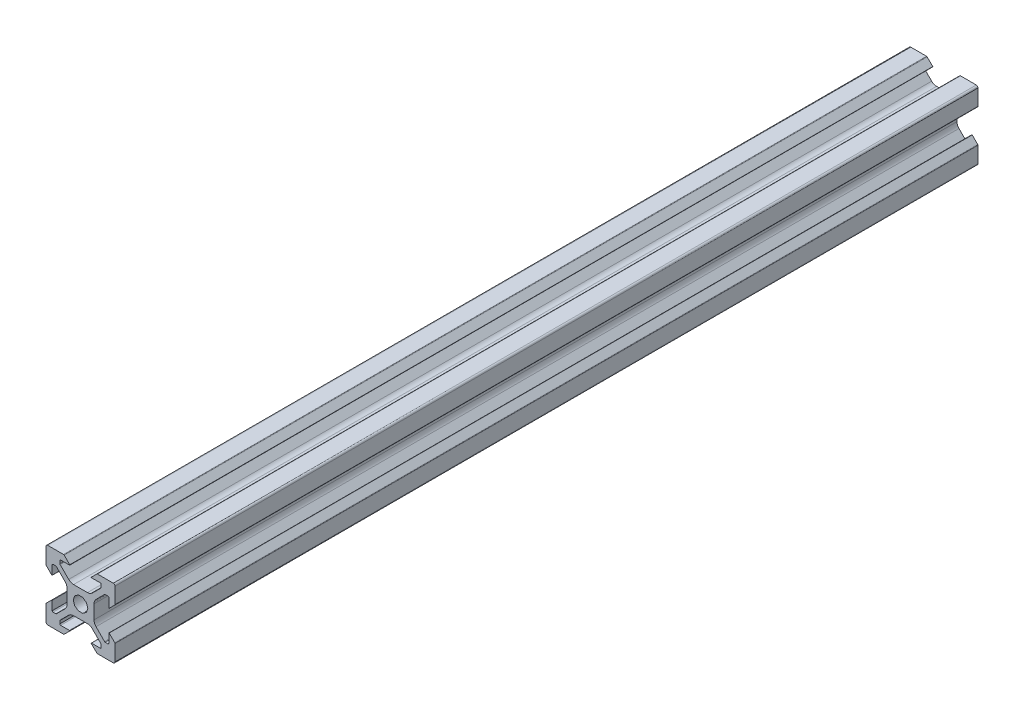
# Autodesk Inventor part: в_профиль 2020
Saved by Autodesk Inventor 2024.2 (Build 282272000, 272)
## iProperties
Created: 2026-01-28
Part Number: в_профиль 2020
Material: Типовые
Document SubType Name: Modeling
Designer: Zakhar
Density: 1 g/cm^3
Appearance: По умолчанию
Author: Zakhar
Autodesk Inventor part; units mm, degrees
ref_plane "YZ Plane" through (0, 0, 0) normal (1, 0, 0) x (0, 1, 0)
ref_plane "XZ Plane" through (0, 0, 0) normal (0, 1, 0) x (-1, 0, 0)
ref_plane "XY Plane" through (0, 0, 0) normal (0, 0, 1) x (1, 0, 0)
ref_plane "РабПлоскость1" through (93.2162, -29.7513, -35.544) normal (0, 0, 1) x (1, 0, 0)
sketch "Эскиз1" plane through (93.2162, -29.7513, -35.544) normal (0, 0, 1) x (1, 0, 0)
  line L0 (3.9, -2.0109) -> (3.9, 2.0109) projected
  arc A0 (4.4858, 3.4251) -> (3.9, 2.0109) centre (5.9, 2.0109) ccw projected
  line L1 (4.4858, 3.4251) -> (6.9874, 5.9268) projected
  arc A1 (7.1642, 6) -> (6.9874, 5.9268) centre (7.1642, 5.75) ccw projected
  line L2 (7.1642, 6) -> (7.95, 6) projected
  arc A2 (8.2, 5.75) -> (7.95, 6) centre (7.95, 5.75) ccw projected
  line L3 (8.2, 5.75) -> (8.2, 3.169) projected
  arc A3 (8.2, 3.169) -> (8.3195, 3.1195) centre (8.27, 3.169) ccw projected
  line L4 (8.3195, 3.1195) -> (9.9268, 4.7268) projected
  arc A4 (9.9268, 4.7268) -> (10, 4.9036) centre (9.75, 4.9036) ccw projected
  line L5 (10, 4.9036) -> (10, 9.5) projected
  arc A5 (10, 9.5) -> (9.5, 10) centre (9.5, 9.5) ccw projected
  line L6 (9.5, 10) -> (4.9036, 10) projected
  arc A6 (4.9036, 10) -> (4.7268, 9.9268) centre (4.9036, 9.75) ccw projected
  line L7 (4.7268, 9.9268) -> (3.1195, 8.3195) projected
  arc A7 (3.1195, 8.3195) -> (3.169, 8.2) centre (3.169, 8.27) ccw projected
  line L8 (3.169, 8.2) -> (5.75, 8.2) projected
  arc A8 (6, 7.95) -> (5.75, 8.2) centre (5.75, 7.95) ccw projected
  line L9 (6, 7.95) -> (6, 7.1642) projected
  arc A9 (5.9268, 6.9874) -> (6, 7.1642) centre (5.75, 7.1642) ccw projected
  line L10 (5.9268, 6.9874) -> (3.4251, 4.4858) projected
  arc A10 (2.0109, 3.9) -> (3.4251, 4.4858) centre (2.0109, 5.9) ccw projected
  line L11 (2.0109, 3.9) -> (-2.0109, 3.9) projected
  arc A11 (-3.4251, 4.4858) -> (-2.0109, 3.9) centre (-2.0109, 5.9) ccw projected
  line L12 (-3.4251, 4.4858) -> (-5.9268, 6.9874) projected
  arc A12 (-6, 7.1642) -> (-5.9268, 6.9874) centre (-5.75, 7.1642) ccw projected
  line L13 (-6, 7.1642) -> (-6, 7.95) projected
  arc A13 (-5.75, 8.2) -> (-6, 7.95) centre (-5.75, 7.95) ccw projected
  line L14 (-5.75, 8.2) -> (-3.169, 8.2) projected
  arc A14 (-3.169, 8.2) -> (-3.1195, 8.3195) centre (-3.169, 8.27) ccw projected
  line L15 (-3.1195, 8.3195) -> (-4.7268, 9.9268) projected
  arc A15 (-4.7268, 9.9268) -> (-4.9036, 10) centre (-4.9036, 9.75) ccw projected
  line L16 (-4.9036, 10) -> (-9.5, 10) projected
  arc A16 (-9.5, 10) -> (-10, 9.5) centre (-9.5, 9.5) ccw projected
  line L17 (-10, 9.5) -> (-10, 4.9036) projected
  arc A17 (-10, 4.9036) -> (-9.9268, 4.7268) centre (-9.75, 4.9036) ccw projected
  line L18 (-9.9268, 4.7268) -> (-8.3195, 3.1195) projected
  arc A18 (-8.3195, 3.1195) -> (-8.2, 3.169) centre (-8.27, 3.169) ccw projected
  line L19 (-8.2, 3.169) -> (-8.2, 5.75) projected
  arc A19 (-7.95, 6) -> (-8.2, 5.75) centre (-7.95, 5.75) ccw projected
  line L20 (-7.95, 6) -> (-7.1642, 6) projected
  arc A20 (-6.9874, 5.9268) -> (-7.1642, 6) centre (-7.1642, 5.75) ccw projected
  line L21 (-6.9874, 5.9268) -> (-4.4858, 3.4251) projected
  arc A21 (-3.9, 2.0109) -> (-4.4858, 3.4251) centre (-5.9, 2.0109) ccw projected
  line L22 (-3.9, 2.0109) -> (-3.9, -2.0109) projected
  arc A22 (-4.4858, -3.4251) -> (-3.9, -2.0109) centre (-5.9, -2.0109) ccw projected
  line L23 (-4.4858, -3.4251) -> (-6.9874, -5.9268) projected
  arc A23 (-7.1642, -6) -> (-6.9874, -5.9268) centre (-7.1642, -5.75) ccw projected
  line L24 (-7.1642, -6) -> (-7.95, -6) projected
  arc A24 (-8.2, -5.75) -> (-7.95, -6) centre (-7.95, -5.75) ccw projected
  line L25 (-8.2, -5.75) -> (-8.2, -3.169) projected
  arc A25 (-8.2, -3.169) -> (-8.3195, -3.1195) centre (-8.27, -3.169) ccw projected
  line L26 (-8.3195, -3.1195) -> (-9.9268, -4.7268) projected
  arc A26 (-9.9268, -4.7268) -> (-10, -4.9036) centre (-9.75, -4.9036) ccw projected
  line L27 (-10, -4.9036) -> (-10, -9.5) projected
  arc A27 (-10, -9.5) -> (-9.5, -10) centre (-9.5, -9.5) ccw projected
  line L28 (-9.5, -10) -> (-4.9036, -10) projected
  arc A28 (-4.9036, -10) -> (-4.7268, -9.9268) centre (-4.9036, -9.75) ccw projected
  line L29 (-4.7268, -9.9268) -> (-3.1195, -8.3195) projected
  arc A29 (-3.1195, -8.3195) -> (-3.169, -8.2) centre (-3.169, -8.27) ccw projected
  line L30 (-3.169, -8.2) -> (-5.75, -8.2) projected
  arc A30 (-6, -7.95) -> (-5.75, -8.2) centre (-5.75, -7.95) ccw projected
  line L31 (-6, -7.95) -> (-6, -7.1642) projected
  arc A31 (-5.9268, -6.9874) -> (-6, -7.1642) centre (-5.75, -7.1642) ccw projected
  line L32 (-5.9268, -6.9874) -> (-3.4251, -4.4858) projected
  arc A32 (-2.0109, -3.9) -> (-3.4251, -4.4858) centre (-2.0109, -5.9) ccw projected
  line L33 (-2.0109, -3.9) -> (2.0109, -3.9) projected
  arc A33 (3.4251, -4.4858) -> (2.0109, -3.9) centre (2.0109, -5.9) ccw projected
  line L34 (3.4251, -4.4858) -> (5.9268, -6.9874) projected
  arc A34 (6, -7.1642) -> (5.9268, -6.9874) centre (5.75, -7.1642) ccw projected
  line L35 (6, -7.1642) -> (6, -7.95) projected
  arc A35 (5.75, -8.2) -> (6, -7.95) centre (5.75, -7.95) ccw projected
  line L36 (5.75, -8.2) -> (3.169, -8.2) projected
  arc A36 (3.169, -8.2) -> (3.1195, -8.3195) centre (3.169, -8.27) ccw projected
  line L37 (3.1195, -8.3195) -> (4.7268, -9.9268) projected
  arc A37 (4.7268, -9.9268) -> (4.9036, -10) centre (4.9036, -9.75) ccw projected
  line L38 (4.9036, -10) -> (9.5, -10) projected
  arc A38 (9.5, -10) -> (10, -9.5) centre (9.5, -9.5) ccw projected
  line L39 (10, -9.5) -> (10, -4.9036) projected
  arc A39 (10, -4.9036) -> (9.9268, -4.7268) centre (9.75, -4.9036) ccw projected
  line L40 (9.9268, -4.7268) -> (8.3195, -3.1195) projected
  arc A40 (8.3195, -3.1195) -> (8.2, -3.169) centre (8.27, -3.169) ccw projected
  line L41 (8.2, -3.169) -> (8.2, -5.75) projected
  arc A41 (7.95, -6) -> (8.2, -5.75) centre (7.95, -5.75) ccw projected
  line L42 (7.95, -6) -> (7.1642, -6) projected
  arc A42 (6.9874, -5.9268) -> (7.1642, -6) centre (7.1642, -5.75) ccw projected
  line L43 (6.9874, -5.9268) -> (4.4858, -3.4251) projected
  arc A43 (3.9, -2.0109) -> (4.4858, -3.4251) centre (5.9, -2.0109) ccw projected
  circle A44 centre (0, 0) radius 2.1 projected
  point P0 (-93.2162, 29.7513)
extrude "Выдавливание1" add sketch "Эскиз1" along normal blind 250
